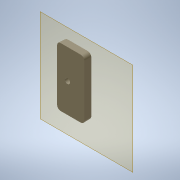
# Autodesk Inventor part: 30_Cube_Z_Focus_MGN_NEMA_counterplate_inner
Saved by Autodesk Inventor 2022 (Build 260153000, 153)
## iProperties
Created: 2021-11-29
Part Number: 30_Cube_Z_Focus_MGN_NEMA_counterplate_inner
Material: Generisch
Document SubType Name: Modeling
Designer: diederichbenedict
Density: 1 g/cm^3
Appearance: Vorgabe
Author: diederichbenedict
Autodesk Inventor part; units mm, degrees
ref_plane "YZ Plane" through (0, 0, 0) normal (1, 0, 0) x (0, 1, 0)
ref_plane "XZ Plane" through (0, 0, 0) normal (0, 1, 0) x (-1, 0, 0)
ref_plane "XY Plane" through (0, 0, 0) normal (0, 0, 1) x (1, 0, 0)
ref_plane "Arbeitsebene1" through (0, 0, 0) normal (0, 0, 1) x (1, 0, 0)
sketch "Skizze1" plane through (0, 0, 0) normal (0, 0, 1) x (1, 0, 0)
  line L0 (20.3781, -18.1328) -> (23.4454, -18.9546) construction
  line L1 (23.4454, -18.9546) -> (24.2672, -22.0219) construction
  line L2 (24.2672, -22.0219) -> (22.0219, -24.2672) construction
  line L3 (22.0219, -24.2672) -> (18.9546, -23.4454) construction
  line L4 (18.9546, -23.4454) -> (18.1328, -20.3781) construction
  line L5 (18.1328, -20.3781) -> (20.3781, -18.1328) construction
  line L6 (-24.2672, 22.0219) -> (-22.0219, 24.2672) construction
  line L7 (-22.0219, 24.2672) -> (-18.9546, 23.4454) construction
  line L8 (-18.9546, 23.4454) -> (-18.1328, 20.3781) construction
  line L9 (-18.1328, 20.3781) -> (-20.3781, 18.1328) construction
  line L10 (-20.3781, 18.1328) -> (-23.4454, 18.9546) construction
  line L11 (-23.4454, 18.9546) -> (-24.2672, 22.0219) construction
  circle A0 centre (20.66, 14.3) radius 2.475 construction
  circle A1 centre (14.3, -20.66) radius 2.475 construction
  circle A2 centre (-20.66, -14.3) radius 2.475 construction
  circle A3 centre (-14.3, 20.66) radius 2.475 construction
  circle A4 centre (14.3, 20.66) radius 2.475 construction
  circle A5 centre (-20.66, 14.3) radius 2.475 construction
  circle A6 centre (-14.3, -20.66) radius 2.475 construction
  circle A7 centre (20.66, -14.3) radius 2.475 construction
  arc A8 (-8.8, -18.96) -> (-8.8, -22.36) centre (-8.8, -20.66) ccw construction
  line L12 (-8.8, -18.96) -> (8.8, -18.96) construction
  arc A9 (8.8, -22.36) -> (8.8, -18.96) centre (8.8, -20.66) ccw construction
  line L13 (8.8, -22.36) -> (-8.8, -22.36) construction
  arc A10 (-8.8, 22.36) -> (-8.8, 18.96) centre (-8.8, 20.66) ccw construction
  line L14 (-8.8, 22.36) -> (8.8, 22.36) construction
  arc A11 (8.8, 18.96) -> (8.8, 22.36) centre (8.8, 20.66) ccw construction
  line L15 (8.8, 18.96) -> (-8.8, 18.96) construction
  arc A12 (-18.96, 8.8) -> (-22.36, 8.8) centre (-20.66, 8.8) ccw construction
  line L16 (-18.96, 8.8) -> (-18.96, -8.8) construction
  arc A13 (-22.36, -8.8) -> (-18.96, -8.8) centre (-20.66, -8.8) ccw construction
  line L17 (-22.36, -8.8) -> (-22.36, 8.8) construction
  arc A14 (18.96, -8.8) -> (22.36, -8.8) centre (20.66, -8.8) ccw construction
  line L18 (18.96, -8.8) -> (18.96, 8.8) construction
  arc A15 (22.36, 8.8) -> (18.96, 8.8) centre (20.66, 8.8) ccw construction
  line L19 (22.36, 8.8) -> (22.36, -8.8) construction
  line L20 (-16.97, -16.97) -> (-16.97, 16.97) construction
  line L21 (-16.97, 16.97) -> (16.97, 16.97) construction
  line L22 (16.97, 16.97) -> (16.97, -16.97) construction
  line L23 (16.97, -16.97) -> (-16.97, -16.97) construction
  circle A16 centre (-21.2, -21.2) radius 2.75 construction
  circle A17 centre (21.2, 21.2) radius 2.75 construction
  arc A18 (-24.35, -22.85) -> (-22.85, -24.35) centre (-22.85, -22.85) ccw construction
  line L24 (22.85, -24.35) -> (-22.85, -24.35) construction
  arc A19 (22.85, -24.35) -> (24.35, -22.85) centre (22.85, -22.85) ccw construction
  line L25 (24.35, 22.85) -> (24.35, -22.85) construction
  arc A20 (24.35, 22.85) -> (22.85, 24.35) centre (22.85, 22.85) ccw construction
  line L26 (-22.85, 24.35) -> (22.85, 24.35) construction
  arc A21 (-22.85, 24.35) -> (-24.35, 22.85) centre (-22.85, 22.85) ccw construction
  line L27 (-24.35, -22.85) -> (-24.35, 22.85) construction
  line L28 (-16.97, 16.97) -> (16.97, 16.97)
  line L29 (16.97, 16.97) -> (16.97, -16.97)
  line L30 (16.97, -16.97) -> (-16.97, -16.97)
  line L31 (-16.97, -16.97) -> (-16.97, 16.97)
  point P0 (0, 0)
  constraints: 8 end point, 2 parallel, 1 horizontal, 1 perpendicular
extrude "Extrusion1" add sketch "Skizze1" against normal blind 4 draft -2
sketch "Skizze2" plane through (0, 0, 0) normal (0, 0, 1) x (1, 0, 0)
  circle A0 centre (-11.03, 0) radius 2.5 projected
  circle A1 centre (-11.03, 0) radius 1.5
  point P0 (0, 0)
  dimension "d3" = 3
  constraints: 1 centre point, 1 coincident
  measures "d3" diameter of A1
extrude "Extrusion2" cut sketch "Skizze2" against normal blind 4 contours A1
fillet "Rundung1" radius 2 4 edges at (-16.9002, -16.9002, -2) (16.9002, -16.9002, -2) (16.9002, 16.9002, -2) (-16.9002, 16.9002, -2)
sketch "Skizze3" plane through (0, 0, 0) normal (0, 0, 1) x (1, 0, 0)
  circle A0 centre (28.0867, -9.6825) radius 1.4 construction
  circle A1 centre (33.0867, 9.6314) radius 1.4 construction
  circle A2 centre (33.0867, -9.6825) radius 1.4 construction
  circle A3 centre (28.0867, 9.6314) radius 1.4 construction
  circle A4 centre (-11.03, 0) radius 3 construction
  circle A5 centre (0.47, 11.5) radius 1.75 construction
  circle A6 centre (0.47, -11.5) radius 1.75 construction
  line L0 (14.4713, 6.5256) -> (36.5731, 6.5256) construction
  line L1 (36.5731, 16.4952) -> (36.5731, 6.5256) construction
  line L2 (-2.8633, 16.4952) -> (36.5731, 16.4952) construction
  line L3 (-24.53, 3.4952) -> (-2.8633, 16.4952) construction
  line L4 (-24.53, 3.4952) -> (-24.53, -3.4952) construction
  line L5 (-24.53, -3.4952) -> (-2.8633, -16.4952) construction
  line L6 (-2.8633, -16.4952) -> (36.5731, -16.4952) construction
  line L7 (36.5731, -16.4952) -> (36.5731, -6.4744) construction
  line L8 (36.5731, -6.4744) -> (14.4713, -6.4744) construction
  line L9 (14.4713, -6.4744) -> (14.4713, -13.5) construction
  line L10 (14.4713, -13.5) -> (4.1713, -13.5) construction
  line L11 (4.1713, -13.5) -> (4.1713, 13.5) construction
  line L12 (4.1713, 13.5) -> (14.4713, 13.5) construction
  line L13 (14.4713, 13.5) -> (14.4713, 6.5256) construction
  circle A7 centre (-11.03, 0) radius 1.5 construction
  ellipse E0 centre (-14.9688, 14.9688) end of major axis (-16.3847, 16.3847) minor radius 2 (-14.9712, 16.97) -> (-16.97, 14.9712) ccw construction
  line L14 (-16.97, 14.9712) -> (-16.97, -14.9712) construction
  ellipse E1 centre (-14.9688, -14.9688) end of major axis (-16.3847, -16.3847) minor radius 2 (-16.97, -14.9712) -> (-14.9712, -16.97) ccw construction
  line L15 (-14.9712, -16.97) -> (14.9712, -16.97) construction
  ellipse E2 centre (14.9688, -14.9688) end of major axis (16.3847, -16.3847) minor radius 2 (14.9712, -16.97) -> (16.97, -14.9712) ccw construction
  line L16 (16.97, -14.9712) -> (16.97, 14.9712) construction
  ellipse E3 centre (14.9688, 14.9688) end of major axis (16.3847, 16.3847) minor radius 2 (16.97, 14.9712) -> (14.9712, 16.97) ccw construction
  line L17 (14.9712, 16.97) -> (-14.9712, 16.97) construction
  line L18 (-14.8315, -16.8303) -> (14.8315, -16.8303) projected
  line L19 (16.97, 16.97) -> (-1.28, 16.97)
  line L20 (-1.28, 16.97) -> (-1.28, -16.8303)
  line L21 (-1.28, -16.8303) -> (16.97, -16.8303)
  line L22 (16.97, -16.8303) -> (16.97, 16.97)
  line L23 (-14.9712, -16.97) -> (14.9712, -16.97) projected
  line L24 (16.97, -16.8303) -> (-1.28, -16.8303)
  line L25 (-1.28, -16.8303) -> (-1.28, -16.97)
  line L26 (-1.28, -16.97) -> (16.97, -16.97)
  line L27 (16.97, -16.97) -> (16.97, -16.8303)
  point P0 (0, 0)
  point P1 (14.8315, -16.8303)
  constraints: 16 end point, 4 parallel, 2 horizontal, 2 perpendicular, 2 point on line, 4 other
extrude "Extrusion3" cut sketch "Skizze3" against normal blind 4
fillet "Rundung2" radius 2 2 edges at (-1.28, -16.9002, -2) (-1.28, 16.9002, -2)
